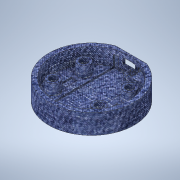
# Autodesk Inventor part: Base
Saved by Autodesk Inventor 2020.1 (Build 241239000, 239)
## iProperties
Created: 2019-10-05
Part Number: Base
Material: Generic
Document SubType Name: Modeling
Designer: Josiah
Density: 1 g/cm^3
Appearance: Denim - Blue
Author: Josiah
Autodesk Inventor part; units mm, degrees
ref_plane "YZ Plane" through (0, 0, 0) normal (1, 0, 0) x (0, 1, 0)
ref_plane "XZ Plane" through (0, 0, 0) normal (0, 1, 0) x (-1, 0, 0)
ref_plane "XY Plane" through (0, 0, 0) normal (0, 0, 1) x (1, 0, 0)
sketch "Sketch1" plane through (0, 0, 0) normal (0, 1, 0) x (-1, 0, 0)
  line L0 (8.5, 21.5) -> (-8.5, 21.5) construction
  line L1 (-8.5, 21.5) -> (-8.5, -21.5) construction
  line L2 (8.5, -21.5) -> (8.5, 21.5) construction
  line L3 (-8.5, 21.5) -> (8.5, -21.5) construction
  line L4 (-8.5, -21.5) -> (8.5, 21.5) construction
  line L5 (-3.5, -21.5) -> (-3.5, -23.5) construction
  line L6 (-3.5, -23.5) -> (3.5, -23.5) construction
  line L7 (3.5, -23.5) -> (3.5, -21.5) construction
  line L8 (-8.5, -21.5) -> (-3.5, -21.5) construction
  line L9 (3.5, -21.5) -> (8.5, -21.5) construction
  arc A0 (9.5253, -23.1034) -> (-9.5253, -23.1034) centre (0, 0) ccw
  line L10 (9.5253, -23.1034) -> (-9.5253, -23.1034)
  line L11 (-10.102, -26.1034) -> (10.102, -26.1034)
  arc A1 (10.102, -26.1034) -> (-10.102, -26.1034) centre (0, 0) ccw
  dimension "d0" = 43
  dimension "d1" = 17
  dimension "d2" = 7
  dimension "d3" = 2
  dimension "d4" = 3
  dimension "d13" = 20.204
  constraints: 24 end point, 4 parallel, 4 point on circle, 2 centre point, 1 coincident, 1 horizontal, 1 perpendicular, 1 other
  measures "d0" distance of L2.start L0.start
  measures "d1" distance of L1.end L2.start
  measures "d2" distance of L5.end L6.end
  measures "d3" distance of L5.start L5.end
  measures "d4" radial gap between concentric circles of A0 A1
  measures "d13" distance of L11.start L11.end
extrude "BASE PLATE" add sketch "Sketch1" along normal blind 3 contours L10 A0 | A1 L11
sketch "Sketch3" plane through (0, 3, 0) normal (0, 1, 0) x (1, 0, 0)
  line L0 (10.102, 26.1034) -> (-10.102, 26.1034) projected
  arc A0 (-10.102, 26.1034) -> (10.102, 26.1034) centre (0, 0) ccw
  arc A1 (-10.102, 26.1034) -> (10.102, 26.1034) centre (0, 0) ccw projected
  line L1 (-10.102, 26.1034) -> (10.102, 26.1034)
  circle A2 centre (0, 0) radius 24.99
  dimension "d58" = 3
  constraints: 4 coincident, 3 end point, 2 centre point, 2 point on circle, 1 collinear, 4 other
  measures "d58" radial gap between concentric circles of A0 A2
extrude "WALLS" add sketch "Sketch3" along normal blind 10
sketch "Sketch6" plane through (0, 3, 0) normal (0, 1, 0) x (1, 0, 0)
  line L0 (-8.5, 21.5) -> (8.5, 21.5) construction
  line L1 (8.5, 21.5) -> (8.5, -21.5) construction
  line L2 (8.5, -21.5) -> (-8.5, -21.5) construction
  line L3 (-8.5, -21.5) -> (-8.5, 21.5) construction
  line L4 (-8.5, -21.5) -> (8.5, 21.5) construction
  line L5 (-8.5, 21.5) -> (8.5, -21.5) construction
  line L6 (0, 0) -> (-15, 0) construction
  line L7 (-15, 0) -> (-15, 10) construction
  line L8 (-15, 10) -> (0, 10) construction
  line L9 (0, 10) -> (0, 0) construction
  circle A0 centre (-15, 10) radius 4
  circle A1 centre (-15, 10) radius 2.5
  circle A2 centre (-15, -10) radius 4
  circle A3 centre (-15, -10) radius 2.5
  circle A4 centre (15, 10) radius 4
  circle A5 centre (15, 10) radius 2.5
  circle A6 centre (15, -10) radius 2.5
  circle A7 centre (15, -10) radius 4
  dimension "d18" = 43
  dimension "d19" = 17
  dimension "d20" = 15
  dimension "d21" = 10
  dimension "d22" = 8
  dimension "d23" = 5
  constraints: 20 end point, 8 centre point, 6 symmetric about line, 5 coincident, 4 parallel, 2 horizontal, 2 perpendicular, 6 other
  measures "d18" distance of L0.end L1.end
  measures "d19" distance of L0.start L0.end
  measures "d20" distance of L7.end L8.end
  measures "d21" distance of L6.end L7.end
  measures "d22" diameter of A0
  measures "d23" diameter of A1
extrude "BUTTON POSTS" add sketch "Sketch6" along normal blind 7
sketch "Sketch7" plane through (0, 3, 0) normal (0, 1, 0) x (1, 0, 0)
  line L0 (-9, 24.1034) -> (9, 24.1034)
  line L1 (9, 24.1034) -> (9, -19.0966)
  line L2 (9, -19.0966) -> (-9, -19.0966)
  line L3 (-9, -19.0966) -> (-9, 24.1034)
  line L4 (-17, 3.75) -> (-13, 3.75)
  line L5 (-13, 3.75) -> (-13, -3.75)
  line L6 (-13, -3.75) -> (-17, -3.75)
  line L7 (-17, -3.75) -> (-17, 3.75)
  line L8 (-24.99, 0) -> (24.99, 0) construction
  line L9 (0, 23.1034) -> (0, -24.99) construction
  line L10 (17, 3.75) -> (13, 3.75)
  line L11 (13, 3.75) -> (13, -3.75)
  line L12 (13, -3.75) -> (17, -3.75)
  line L13 (17, -3.75) -> (17, 3.75)
  line L14 (-9.5253, 24.1034) -> (9.5253, 24.1034) projected
  line L15 (10.102, 26.1034) -> (-10.102, 26.1034) projected
  dimension "d26" = 43.2
  dimension "d27" = 18
  dimension "d28" = 7.5
  dimension "d29" = 4
  dimension "d30" = 3.75
  dimension "d63" = 2
  dimension "d65" = 9
  dimension "d77" = 13
  constraints: 28 end point, 4 horizontal, 4 parallel, 4 symmetric about line, 2 perpendicular, 1 vertical
  measures "d26" distance of L2.end L0.start
  measures "d27" distance of L0.start L0.end
  measures "d28" distance of L4.end L5.end
  measures "d29" distance of L4.start L4.end
  measures "d30" distance between parallel lines of L4 L8
  measures "d63" distance between parallel lines of L0 L15
  measures "d65" distance between parallel lines of L9 L3
  measures "d77" distance between parallel lines of L5 L9
extrude "INDENTATION FOR LINEUP" cut sketch "Sketch7" against normal blind 1
sketch "Sketch9" plane through (0, 2, 0) normal (0, 1, 0) x (1, 0, 0)
  line L0 (-9, 24.1034) -> (9, 24.1034) projected
  line L1 (-9, -19.0966) -> (9, -19.0966)
  line L2 (9, -19.0966) -> (9, 24.1034)
  line L3 (9, 24.1034) -> (-9, 24.1034)
  line L4 (-9, 24.1034) -> (-9, -19.0966)
  point P0 (0, 0)
  constraints: 8 end point, 2 parallel, 1 horizontal, 1 perpendicular
extrude "FLAT SURFACE FOR ARDUINO" cut sketch "Sketch9" along normal blind 8
sketch "Sketch12" plane through (0, 3, 0) normal (0, 1, 0) x (1, 0, 0)
  line L0 (19.1097, 16.1034) -> (9, 16.1034)
  line L1 (9, 16.1034) -> (9, 23.3131)
  line L2 (-9, 24.1034) -> (9, 24.1034) construction
  line L3 (-9, -19.0966) -> (-9, 24.1034) construction
  line L4 (9, -19.0966) -> (-9, -19.0966) construction
  line L5 (9, 24.1034) -> (9, -19.0966) construction
  line L6 (10.102, 26.1034) -> (-10.102, 26.1034) projected
  circle A0 centre (0, 0) radius 24.99 construction
  arc A1 (-9, 23.3131) -> (9, 23.3131) centre (0, 0) ccw projected
  arc A2 (19.1097, 16.1034) -> (9, 23.3131) centre (0, 0) ccw
  line L7 (9, 23.3131) -> (9, -19.0966) projected
  point P0 (13, 21.3424)
  dimension "d88" = 10
  constraints: 4 end point, 4 point on circle, 1 centre point, 1 coincident, 1 collinear, 1 concentric, 1 horizontal, 1 point on line, 1 vertical, 4 other
  measures "d88" distance between parallel lines of L6 L0
extrude "PIN SUPPORT TOWER" add sketch "Sketch12" along normal blind 7
sketch "Sketch16" plane through (9, 2, -24.1034) normal (-1, 0, 0) x (0, 0, 1)
  line L0 (0.7903, 8) -> (8, 8) construction
  line L1 (6, 8) -> (6, 5.7) construction
  line L2 (6, 5.7) -> (4.3, 5.7) construction
  line L3 (4.3, 5.7) -> (4.3, 8) construction
  line L4 (0.7903, 8) -> (8, 8) construction
  line L5 (8, 1) -> (8, 8) construction
  line L6 (0.7903, 8) -> (8, 8) construction
  line L7 (14.8538, 7.25) -> (0, 7.25) construction
  line L8 (0, 0) -> (0, 8) construction
  line L9 (3, 8) -> (8, 8)
  line L10 (8, 8) -> (8, 5)
  line L11 (8, 5) -> (3, 5)
  line L12 (3, 5) -> (3, 8)
  point P0 (24.1034, -2)
  dimension "d96" = 3
  dimension "d97" = 5
  constraints: 10 end point, 2 horizontal, 2 parallel, 1 perpendicular, 1 point on line
  measures "d96" distance of L0.end L10.end
  measures "d97" distance of L0.end L9.start
extrude "PIN SUPPORT BEAM" add sketch "Sketch16" along normal blind 4.398
sketch "Sketch18" plane through (0, 10, 0) normal (0, 1, 0) x (1, 0, 0)
  line L0 (9.727, 18.1034) -> (5.477, 18.1034)
  line L1 (5.477, 18.1034) -> (5.477, 20.1034)
  line L2 (5.477, 20.1034) -> (9.727, 20.1034)
  line L3 (9.727, 20.1034) -> (9.727, 18.1034)
  line L4 (19.1097, 16.1034) -> (4.602, 16.1034) projected
  line L5 (4.602, 16.1034) -> (4.602, 21.1034) projected
  line L6 (8.468, 23.5115) -> (8.468, 24.1034) projected
  line L7 (6.736, 24.1034) -> (6.736, 24.065) projected
  line L8 (8.468, 24.1034) -> (6.736, 24.1034) projected
  line L9 (6.602, 26.1034) -> (8.602, 26.1034) projected
  line L10 (7.602, 26.1034) -> (7.602, 13.109) construction
  point P0 (0, 0)
  dimension "d104" = 2
  dimension "d105" = 4.25
  dimension "d106" = 2
  dimension "d108" = 2.125
  constraints: 10 end point, 2 parallel, 1 horizontal, 1 midpoint, 1 perpendicular, 1 vertical, 1 other
  measures "d104" distance between parallel lines of L4 L0
  measures "d105" distance between parallel lines of L3 L1
  measures "d106" distance of L2.end L0.start
  measures "d108" distance between parallel lines of L3 L10
extrude "M2 NUT HOLDER" cut sketch "Sketch18" against normal blind 2.3
sketch "Sketch20" plane through (0, 7.7, 0) normal (0, 1, 0) x (1, 0, 0)
  line L0 (9, 24.1034) -> (9, -19.0966) projected
  line L1 (5.477, 20.1034) -> (9.727, 20.1034) projected
  line L2 (5.477, 18.1034) -> (5.477, 20.1034) projected
  line L3 (9, 16.1034) -> (9, 21.1034) projected
  line L4 (9, 20.1034) -> (5.477, 20.1034)
  line L5 (5.477, 20.1034) -> (5.477, 18.1034)
  line L6 (5.477, 18.1034) -> (9, 18.1034)
  line L7 (9, 18.1034) -> (9, 20.1034)
  point P0 (0, 0)
  constraints: 8 end point, 2 parallel, 2 point on line, 1 horizontal, 1 perpendicular
extrude "M2 PASS-THROUGH HOLE" cut sketch "Sketch20" against normal up to next
sketch "Sketch11" plane through (10.102, 0, -26.1034) normal (0, 0, -1) x (-1, 0, 0)
  line L0 (19.102, 2) -> (1.102, 2) construction
  line L1 (0, 0) -> (0, 13) construction
  line L2 (20.204, 0) -> (20.204, 13) construction
  line L3 (6.1, 10) -> (14.1, 10)
  line L4 (14.1, 10) -> (14.1, 6)
  line L5 (14.1, 6) -> (6.1, 6)
  line L6 (6.1, 6) -> (6.1, 10)
  line L7 (0, 0) -> (20.204, 0) construction
  circle A0 centre (2.5, 9.5) radius 1
  point P0 (10.102, 0)
  dimension "d69" = 4
  dimension "d70" = 4
  dimension "d71" = 6.1
  dimension "d72" = 2
  dimension "d74" = 2.5
  dimension "d78" = 7.5
  dimension "d89" = 8
  constraints: 8 end point, 2 parallel, 1 centre point, 1 horizontal, 1 perpendicular
  measures "d69" distance of L3.end L4.end
  measures "d70" distance between parallel lines of L5 L0
  measures "d71" distance between parallel lines of L1 L6
  measures "d72" diameter of A0
  measures "d74" distance from line of L1 A0.centre
  measures "d78" distance from line of A0.centre L0
  measures "d89" distance of L3.start L3.end
extrude "I/O HOLES" cut sketch "Sketch11" against normal blind 15
fillet "SMOOTHING M2 NUT HOLDER" radius 1 7 edges at (8.468, 10, -20.6034) (6.736, 10, -17.1034) (8.468, 10, -17.1034) (6.736, 10, -20.6034) (4.602, 7, -18.6034) (9, 7, -17.1034) (9, 7, -20.6034)
sketch "Sketch21" plane through (0, 0, 0) normal (0, -1, 0) x (1, 0, 0)
  line L0 (20.0639, 17.6764) -> (20.0639, -57.2384) construction
  line L1 (20.0639, -57.2384) -> (13.2865, -57.2384) construction
  line L2 (13.2865, -57.2384) -> (13.2865, 17.6764) construction
  line L3 (13.2865, 17.6764) -> (20.0639, 17.6764) construction
  spline S0 degree 2 poles (15.339, 13.7944) (14.9176, 13.7944) (14.1697, 14.0841) (13.9063, 14.3738) knots 0 0 0 1 2 2 2
  spline S1 degree 2 poles (13.9063, 14.3738) (13.6113, 14.7004) (13.3321, 15.5905) (13.3321, 16.17) knots 0 0 0 1 2 2 2
  spline S2 degree 2 poles (13.3321, 16.17) (13.3321, 16.6019) (13.3954, 17.3604) (13.4586, 17.6501) knots 0 0 0 1 2 2 2
  line L4 (13.4586, 17.6501) -> (14.7754, 17.6501)
  line L5 (14.7754, 17.6501) -> (14.7754, 17.5026)
  spline S3 degree 2 poles (14.7754, 17.5026) (14.6964, 17.3077) (14.5595, 16.8811) (14.5595, 16.544) knots 0 0 0 1 2 2 2
  spline S4 degree 2 poles (14.5595, 16.544) (14.5595, 16.112) (14.8018, 15.6432) (15.023, 15.5484) knots 0 0 0 1 2 2 2
  spline S5 degree 2 poles (15.023, 15.5484) (15.239, 15.4483) (15.7973, 15.4273) (16.145, 15.4273) knots 0 0 0 1 2 2 2
  line L6 (16.145, 15.4273) -> (18.7523, 15.4273)
  line L7 (18.7523, 15.4273) -> (18.7523, 16.9127)
  line L8 (18.7523, 16.9127) -> (19.9322, 16.9127)
  line L9 (19.9322, 16.9127) -> (19.9322, 13.7944)
  line L10 (19.9322, 13.7944) -> (15.339, 13.7944)
  spline S6 degree 2 poles (15.4233, 7.3365) (14.9387, 7.3365) (14.2065, 7.7052) (13.9642, 8.0107) knots 0 0 0 1 2 2 2
  spline S7 degree 2 poles (13.9642, 8.0107) (13.6745, 8.3794) (13.4322, 9.2538) (13.4322, 9.9333) knots 0 0 0 1 2 2 2
  line L11 (13.4322, 9.9333) -> (13.4322, 12.5302)
  line L12 (13.4322, 12.5302) -> (19.9322, 12.5302)
  line L13 (19.9322, 12.5302) -> (19.9322, 10.2388)
  spline S8 degree 2 poles (19.9322, 10.2388) (19.9322, 9.5225) (19.8216, 8.785) (19.6478, 8.4637) knots 0 0 0 1 2 2 2
  spline S9 degree 2 poles (19.6478, 8.4637) (19.4634, 8.1108) (18.8313, 7.7684) (18.4205, 7.7684) knots 0 0 0 1 2 2 2
  spline S10 degree 2 poles (18.4205, 7.7684) (17.9464, 7.7684) (17.2037, 8.2425) (17.0299, 8.6639) knots 0 0 0 1 2 2 2
  line L14 (17.0299, 8.6639) -> (16.9983, 8.6639)
  spline S11 degree 2 poles (16.9983, 8.6639) (16.8719, 8.0581) (16.087, 7.3365) (15.4233, 7.3365) knots 0 0 0 1 2 2 2
  spline S12 degree 2 poles (15.4497, 9.0221) (15.7552, 9.0221) (16.0975, 9.2644) (16.1871, 9.5067) knots 0 0 0 1 2 2 2
  spline S13 degree 2 poles (16.1871, 9.5067) (16.245, 9.6542) (16.2556, 10.1756) (16.2556, 10.6076) knots 0 0 0 1 2 2 2
  line L15 (16.2556, 10.6076) -> (16.2556, 10.9078)
  line L16 (16.2556, 10.9078) -> (14.6174, 10.9078)
  line L17 (14.6174, 10.9078) -> (14.6174, 10.8183)
  spline S14 degree 2 poles (14.6174, 10.8183) (14.6174, 10.1862) (14.6332, 9.7016) (14.7438, 9.4487) knots 0 0 0 1 2 2 2
  spline S15 degree 2 poles (14.7438, 9.4487) (14.8439, 9.2275) (15.2126, 9.0221) (15.4497, 9.0221) knots 0 0 0 1 2 2 2
  spline S16 degree 2 poles (18.0992, 9.4277) (18.2572, 9.4277) (18.589, 9.591) (18.6628, 9.7595) knots 0 0 0 1 2 2 2
  spline S17 degree 2 poles (18.6628, 9.7595) (18.7365, 9.9175) (18.7471, 10.36) (18.7471, 10.7972) knots 0 0 0 1 2 2 2
  line L18 (18.7471, 10.7972) -> (18.7471, 10.9078)
  line L19 (18.7471, 10.9078) -> (17.367, 10.9078)
  line L20 (17.367, 10.9078) -> (17.367, 10.7024)
  spline S18 degree 2 poles (17.367, 10.7024) (17.367, 10.2863) (17.3828, 9.9491) (17.4671, 9.77) knots 0 0 0 1 2 2 2
  spline S19 degree 2 poles (17.4671, 9.77) (17.5619, 9.5752) (17.8832, 9.4277) (18.0992, 9.4277) knots 0 0 0 1 2 2 2
  line L21 (13.4322, -0.9808) -> (13.4322, 3.7968)
  line L22 (13.4322, 3.7968) -> (14.491, 3.7968)
  spline S20 degree 2 poles (14.491, 3.7968) (14.9756, 3.191) (15.8289, 2.2218) (16.2134, 1.8584) knots 0 0 0 1 2 2 2
  spline S21 degree 2 poles (16.2134, 1.8584) (16.7138, 1.379) (17.4776, 0.9524) (17.8779, 0.9524) knots 0 0 0 1 2 2 2
  spline S22 degree 2 poles (17.8779, 0.9524) (18.3309, 0.9524) (18.8155, 1.4949) (18.8155, 1.9795) knots 0 0 0 1 2 2 2
  spline S23 degree 2 poles (18.8155, 1.9795) (18.8155, 2.2271) (18.6944, 2.6696) (18.5996, 2.8961) knots 0 0 0 1 2 2 2
  spline S24 degree 2 poles (18.5996, 2.8961) (18.4995, 3.1173) (18.2888, 3.4333) (18.2361, 3.5123) knots 0 0 0 1 2 2 2
  line L23 (18.2361, 3.5123) -> (18.2361, 3.6388)
  line L24 (18.2361, 3.6388) -> (19.6531, 3.6388)
  spline S25 degree 2 poles (19.6531, 3.6388) (19.7847, 3.3649) (20.0586, 2.1955) (20.0586, 1.6529) knots 0 0 0 1 2 2 2
  spline S26 degree 2 poles (20.0586, 1.6529) (20.0586, 0.4941) (19.0262, -0.6963) (18.0939, -0.6963) knots 0 0 0 1 2 2 2
  spline S27 degree 2 poles (18.0939, -0.6963) (17.5197, -0.6963) (16.4136, -0.1538) (15.7815, 0.473) knots 0 0 0 1 2 2 2
  spline S28 degree 2 poles (15.7815, 0.473) (15.3917, 0.8681) (14.786, 1.6108) (14.6595, 1.7741) knots 0 0 0 1 2 2 2
  line L25 (14.6595, 1.7741) -> (14.6595, -0.9808)
  line L26 (14.6595, -0.9808) -> (13.4322, -0.9808)
  spline S29 degree 2 poles (16.6822, -6.5906) (15.8394, -6.5906) (14.5753, -6.3219) (14.1486, -6.0217) knots 0 0 0 1 2 2 2
  spline S30 degree 2 poles (14.1486, -6.0217) (13.7272, -5.7267) (13.2953, -4.7733) (13.2953, -4.0885) knots 0 0 0 1 2 2 2
  spline S31 degree 2 poles (13.2953, -4.0885) (13.2953, -3.3985) (13.7272, -2.4504) (14.1591, -2.1501) knots 0 0 0 1 2 2 2
  spline S32 degree 2 poles (14.1591, -2.1501) (14.5858, -1.8499) (15.8394, -1.5812) (16.6822, -1.5812) knots 0 0 0 1 2 2 2
  spline S33 degree 2 poles (16.6822, -1.5812) (17.5461, -1.5812) (18.7681, -1.8499) (19.2106, -2.1554) knots 0 0 0 1 2 2 2
  spline S34 degree 2 poles (19.2106, -2.1554) (19.6425, -2.4609) (20.0639, -3.4248) (20.0639, -4.0885) knots 0 0 0 1 2 2 2
  spline S35 degree 2 poles (20.0639, -4.0885) (20.0639, -4.7891) (19.6215, -5.7267) (19.1843, -6.027) knots 0 0 0 1 2 2 2
  spline S36 degree 2 poles (19.1843, -6.027) (18.7576, -6.3219) (17.4987, -6.5906) (16.6822, -6.5906) knots 0 0 0 1 2 2 2
  spline S37 degree 2 poles (16.6822, -4.9524) (17.8885, -4.9524) (18.8629, -4.5573) (18.8629, -4.0885) knots 0 0 0 1 2 2 2
  spline S38 degree 2 poles (18.8629, -4.0885) (18.8629, -3.6197) (17.8885, -3.2194) (16.677, -3.2194) knots 0 0 0 1 2 2 2
  spline S39 degree 2 poles (16.677, -3.2194) (15.4865, -3.2194) (14.4962, -3.6197) (14.4962, -4.0885) knots 0 0 0 1 2 2 2
  spline S40 degree 2 poles (14.4962, -4.0885) (14.4962, -4.5521) (15.4865, -4.9524) (16.6822, -4.9524) knots 0 0 0 1 2 2 2
  line L27 (13.4322, -12.0792) -> (13.4322, -7.7863)
  line L28 (13.4322, -7.7863) -> (14.5647, -7.7863)
  line L29 (14.5647, -7.7863) -> (14.5647, -9.1558)
  line L30 (14.5647, -9.1558) -> (18.0044, -9.1558)
  line L31 (18.0044, -9.1558) -> (18.0044, -7.7863)
  line L32 (18.0044, -7.7863) -> (19.0631, -7.7863)
  spline S41 degree 2 poles (19.0631, -7.7863) (19.0631, -8.0865) (19.1421, -8.6817) (19.2264, -8.8608) knots 0 0 0 1 2 2 2
  spline S42 degree 2 poles (19.2264, -8.8608) (19.3317, -9.0663) (19.6847, -9.298) (19.948, -9.3191) knots 0 0 0 1 2 2 2
  line L33 (19.948, -9.3191) -> (19.948, -10.7413)
  line L34 (19.948, -10.7413) -> (14.5647, -10.7413)
  line L35 (14.5647, -10.7413) -> (14.5647, -12.0792)
  line L36 (14.5647, -12.0792) -> (13.4322, -12.0792)
  spline S43 degree 2 poles (17.0457, -17.8945) (16.2187, -17.8945) (14.8386, -17.5099) (14.3435, -17.1043) knots 0 0 0 1 2 2 2
  spline S44 degree 2 poles (14.3435, -17.1043) (13.8431, -16.683) (13.3058, -15.4398) (13.3058, -14.5338) knots 0 0 0 1 2 2 2
  spline S45 degree 2 poles (13.3058, -14.5338) (13.3058, -14.2283) (13.3848, -13.5646) (13.4164, -13.454) knots 0 0 0 1 2 2 2
  line L37 (13.4164, -13.454) -> (14.6911, -13.454)
  line L38 (14.6911, -13.454) -> (14.6911, -13.5804)
  spline S46 degree 2 poles (14.6911, -13.5804) (14.6279, -13.7016) (14.491, -14.1546) (14.491, -14.5496) knots 0 0 0 1 2 2 2
  spline S47 degree 2 poles (14.491, -14.5496) (14.491, -14.871) (14.6595, -15.4662) (14.8439, -15.6769) knots 0 0 0 1 2 2 2
  spline S48 degree 2 poles (14.8439, -15.6769) (15.0388, -15.9034) (15.6129, -16.1983) (16.0449, -16.251) knots 0 0 0 1 2 2 2
  spline S49 degree 2 poles (16.0449, -16.251) (15.8289, -15.9034) (15.5971, -15.3029) (15.5971, -14.8552) knots 0 0 0 1 2 2 2
  spline S50 degree 2 poles (15.5971, -14.8552) (15.5971, -14.5233) (15.7762, -13.907) (15.9659, -13.6542) knots 0 0 0 1 2 2 2
  spline S51 degree 2 poles (15.9659, -13.6542) (16.224, -13.3171) (17.0509, -12.922) (17.7041, -12.922) knots 0 0 0 1 2 2 2
  spline S52 degree 2 poles (17.7041, -12.922) (18.215, -12.922) (19.0736, -13.2697) (19.3897, -13.5857) knots 0 0 0 1 2 2 2
  spline S53 degree 2 poles (19.3897, -13.5857) (19.7057, -13.9018) (20.0639, -14.8183) (20.0639, -15.3819) knots 0 0 0 1 2 2 2
  spline S54 degree 2 poles (20.0639, -15.3819) (20.0639, -15.9508) (19.7479, -16.8304) (19.416, -17.1465) knots 0 0 0 1 2 2 2
  spline S55 degree 2 poles (19.416, -17.1465) (19.0473, -17.5152) (17.8779, -17.8945) (17.0457, -17.8945) knots 0 0 0 1 2 2 2
  spline S56 degree 2 poles (17.288, -16.2774) (17.82, -16.2774) (18.5048, -16.0983) (18.6944, -15.935) knots 0 0 0 1 2 2 2
  spline S57 degree 2 poles (18.6944, -15.935) (18.8366, -15.8244) (18.9578, -15.5399) (18.9578, -15.3766) knots 0 0 0 1 2 2 2
  spline S58 degree 2 poles (18.9578, -15.3766) (18.9578, -15.2291) (18.8419, -14.9552) (18.6944, -14.8288) knots 0 0 0 1 2 2 2
  spline S59 degree 2 poles (18.6944, -14.8288) (18.568, -14.7182) (18.0781, -14.5602) (17.7884, -14.5602) knots 0 0 0 1 2 2 2
  spline S60 degree 2 poles (17.7884, -14.5602) (17.4723, -14.5602) (17.0668, -14.7235) (16.9456, -14.8604) knots 0 0 0 1 2 2 2
  spline S61 degree 2 poles (16.9456, -14.8604) (16.8244, -15.0026) (16.7296, -15.3556) (16.7296, -15.5768) knots 0 0 0 1 2 2 2
  spline S62 degree 2 poles (16.7296, -15.5768) (16.7296, -15.7612) (16.8297, -16.1457) (16.8824, -16.2668) knots 0 0 0 1 2 2 2
  spline S63 degree 2 poles (16.8824, -16.2668) (16.9298, -16.2668) (17.1089, -16.2774) (17.288, -16.2774) knots 0 0 0 1 2 2 2
  point P0 (0, 0)
  constraints: 2 other
emboss "NAME TEXT" sketch "Sketch21" operation cut depth 1 direction (0, 1, 0)
equation "\"d30\" = 0.5 * d28"
equation "\"d65\" = 0.5 * d27"
equation "\"d108\" = 0.5 * d105"
body "Solid1"
